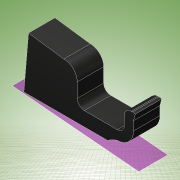
# Autodesk Inventor part: wall_hook
Saved by Autodesk Inventor 2017 (Build 210142000, 142)
## iProperties
Created: 2018-06-04
Part Number: wall_hook
Material: Generic
Document SubType Name: Modeling
Designer: Spark Electronics
Density: 1 g/cm^3
Appearance: Glossy - Black
Author: Spark Electronics
Autodesk Inventor part; units mm, degrees
ref_plane "YZ Plane" through (0, 0, 0) normal (1, 0, 0) x (0, 1, 0)
ref_plane "XZ Plane" through (0, 0, 0) normal (0, 1, 0) x (-1, 0, 0)
ref_plane "XY Plane" through (0, 0, 0) normal (0, 0, 1) x (1, 0, 0)
sketch "Sketch1" plane through (0, 0, 0) normal (0, 0, 1) x (1, 0, 0)
  line L0 (16.6994, 1.0131) -> (16.6994, -5.3643)
  line L1 (11.6194, -10.4443) -> (-12.1882, -10.4443)
  line L2 (-17.2682, -5.3643) -> (-17.2682, 4.9632)
  line L3 (0, -15.049) -> (0, 10.4443)
  arc A0 (-17.2682, -5.3643) -> (-12.1882, -10.4443) centre (-12.1882, -5.3643) ccw
  arc A1 (11.6194, -10.4443) -> (16.6994, -5.3643) centre (11.6194, -5.3643) ccw
  line L4 (21.7794, 6.0931) -> (22.6586, 6.0931)
  line L5 (16.6994, -4.0396) -> (16.6994, 1.0131)
  arc A2 (21.7794, 6.0931) -> (16.6994, 1.0131) centre (21.7794, 1.0131) ccw
  line L6 (26.4264, -0.0507) -> (26.4501, 0)
  arc A3 (24.5947, 5.7097) -> (22.6586, 6.0931) centre (22.6586, 1.0131) ccw
  line L7 (4.7625, -20.6375) -> (-55.8182, -20.6375)
  line L8 (-52.4441, 17.9282) -> (-26.9554, 14.412)
  arc A4 (11.6194, -17.1294) -> (23.3845, -5.3643) centre (11.6194, -5.3643) ccw
  line L9 (23.3845, -5.3643) -> (23.3845, 1.0131)
  line L10 (23.3845, 1.0131) -> (24.5947, 5.7097)
  arc A5 (11.6194, -17.1294) -> (4.7625, -20.6375) centre (16.7372, -35.5878) ccw
  arc A6 (-17.2682, 4.9632) -> (-26.9554, 14.412) centre (-26.7199, 4.9632) ccw
  line L11 (-52.4441, 17.9282) -> (-55.8182, -20.6375)
  point P0 (0, 0)
  dimension "d2" = 5.08
  dimension "d3" = 5.08
  dimension "d6" = 5
  constraints: 24 end point, 14 point on circle, 8 tangent, 7 centre point, 2 horizontal, 1 equal radius, 1 parallel, 1 point on line, 1 vertical, 1 other
  measures "d2" radius of A0
  measures "d3" radius of A2
  measures "d6" angle of L3 L11
extrude "Extrusion1" add sketch "Sketch1" along normal blind 19.05
ref_plane "Work Plane1" through (-55.8182, -20.6375, 0) normal (-0.0871557, -0.9961947, 0) x (0, 0, 1)
sketch "Sketch2" plane through (-55.8182, -20.6375, 0) normal (-0.0871557, -0.9961947, 0) x (0, 0, 1)
  line L0 (19.05, 0) -> (19.05, -60.3501) projected
  line L1 (0, -60.3501) -> (0, 0) projected
  line L2 (15.875, -6.7) -> (13.3103, -1.2)
  line L3 (3.175, -6.7) -> (5.7397, -1.2)
  line L4 (3.175, -6.7) -> (15.875, -6.7)
  line L5 (13.3103, 0.8) -> (5.7397, 0.8)
  line L6 (5.7397, -1.2) -> (5.7397, 0.8)
  line L7 (13.3103, -1.2) -> (13.3103, 0.8)
  line L8 (5.9397, 0.6) -> (13.1103, 0.6)
  line L9 (13.1103, 0.6) -> (13.1103, -1.2443)
  line L10 (13.1103, -1.2443) -> (15.5611, -6.5)
  line L11 (15.5611, -6.5) -> (3.4889, -6.5)
  line L12 (3.4889, -6.5) -> (5.9397, -1.2443)
  line L13 (5.9397, -1.2443) -> (5.9397, 0.6)
  line L14 (9.1778, 2.6147) -> (9.1778, -9.4246) construction
  point P0 (0, -53.8071)
  point P1 (2.5747, 0)
  point P2 (2.5747, 0)
  dimension "d27" = 12.7
  dimension "d28" = 5.5
  dimension "d29" = 5.5
  dimension "d30" = 2
  dimension "d31" = 2
  dimension "d32" = 0.2
  dimension "d33" = 155
  dimension "d34" = 155
  dimension "d35" = 3.175
  constraints: 26 end point, 2 parallel, 2 perpendicular, 1 horizontal, 1 vertical, 5 other
  measures "d27" distance of L3.start L2.start
  measures "d28" distance from line of L4 L6.start
  measures "d29" distance from line of L4 L7.start
  measures "d30" distance of L6.start L6.end
  measures "d31" distance of L7.start L7.end
  measures "d32" distance between parallel lines of L6 L13
  measures "d33" angle of L3 L6
  measures "d34" angle of L2 L7
  measures "d35" distance from line of L3.start L1
extrude "Extrusion2" cut sketch "Sketch2" against normal blind 25.4 contours L4 L3 L6 L5 L7 L2 | L8 L9 L10 L11 L12 L13
body "Solid1"
